servo_mount_post (Autodesk Fusion 360 design; units mm, degrees)
Autodesk Fusion 360 part; units mm, degrees
sketch "Sketch1" plane through (0, 0, 0) normal (0, 0, 1) x (1, 0, 0)
  line L0 (0, 0) -> (23.3, 0)
  line L1 (23.3, 0) -> (23.3, 12.5)
  line L2 (23.3, 12.5) -> (0, 12.5)
  line L3 (0, 12.5) -> (0, 0)
  line L4 (0, 12.5) -> (9.1, 12.5)
  line L5 (9.1, 12.5) -> (9.1, 21.6)
  line L6 (9.1, 21.6) -> (0, 21.6)
  line L7 (0, 21.6) -> (0, 12.5)
  line L8 (9.1, 12.5) -> (11.1, 12.5)
  line L9 (11.1, 12.5) -> (11.1, 17)
  line L10 (11.1, 17) -> (9.1, 17)
  line L11 (9.1, 17) -> (9.1, 12.5)
  line L12 (0, 6.25) -> (23.3, 6.25) construction
  line L13 (23.3, 6.25) -> (25.65, 6.25) construction
  line L14 (0, 6.25) -> (-2.35, 6.25) construction
  circle A0 centre (25.65, 6.25) radius 1.45
  circle A1 centre (-2.35, 6.25) radius 1.45
  line L15 (-5.8, -2) -> (29.1, -2)
  line L16 (29.1, -2) -> (29.1, 23.6)
  line L17 (29.1, 23.6) -> (-5.8, 23.6)
  line L18 (-5.8, 23.6) -> (-5.8, -2)
  dimension "d1" = 23.3
  dimension "d2" = 12.5
  dimension "d3" = 9.1
  dimension "d4" = 9.1
  dimension "d5" = 2
  dimension "d6" = 4.5
  dimension "d7" = 2.35
  dimension "d8" = 2.35
  dimension "d9" = 2.9
  dimension "d10" = 2.9
  dimension "d11" = 3.45
  dimension "d12" = 3.45
  dimension "d13" = 2
  dimension "d14" = 2
  constraint horizontal L0
  constraint vertical L1
  constraint horizontal L2
  constraint vertical L3
  constraint coincident L0.start L3.end
  constraint horizontal L4
  constraint vertical L5
  constraint horizontal L6
  constraint vertical L7
  constraint horizontal L8
  constraint vertical L9
  constraint horizontal L10
  constraint vertical L11
  constraint midpoint L3 L12.start
  constraint midpoint L1 L12.end
  constraint perpendicular L1 L13
  constraint perpendicular L3 L14
  constraint coincident L13.end A0.centre
  constraint coincident L14.end A1.centre
  constraint horizontal L15
  constraint vertical L16
  constraint horizontal L17
  constraint vertical L18
  measures "d1" distance of L0.start L0.end
  measures "d2" distance of L0.start L2.end
  measures "d3" distance of L2.end L4.end
  measures "d4" distance of L2.end L6.end
  measures "d5" distance of L4.end L8.end
  measures "d6" distance of L4.end L10.end
  measures "d7" distance of L12.end L13.end
  measures "d8" distance of L12.start L14.end
  measures "d9" diameter of A0
  measures "d10" diameter of A1
  measures "d11" distance of L14.end L18
  measures "d12" distance of L13.end L16
  measures "d13" distance of L6 L17
  measures "d14" distance of L0 L15
extrude "Extrude1" add sketch "Sketch1" along normal blind 2
sketch "Sketch2" plane through (0, 0, 2) normal (0, 0, 1) x (-1, 0, 0)
  line L0 (-9.1, -17) -> (-11.1, -17)
  line L1 (-11.1, -17) -> (-11.1, -12.5)
  line L2 (-11.1, -12.5) -> (-23.3, -12.5)
  line L3 (-23.3, -12.5) -> (-23.3, 0)
  line L4 (-23.3, 0) -> (0, 0)
  line L5 (0, 0) -> (0, -21.6)
  line L6 (0, -21.6) -> (-9.1, -21.6)
  line L7 (-9.1, -21.6) -> (-9.1, -17)
  circle A0 centre (2.35, -6.25) radius 1.45
  circle A1 centre (-25.65, -6.25) radius 1.45
  line L8 (5.8, -23.6) -> (5.8, 2)
  line L9 (5.8, 2) -> (-29.1, 2)
  line L10 (-29.1, 2) -> (-29.1, -23.6)
  line L11 (-29.1, -23.6) -> (5.8, -23.6)
